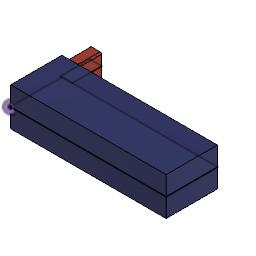
LiPo (Autodesk Fusion 360 design; units mm, degrees)
part number: 2026-02-11-13-17-56-255
Autodesk Fusion 360 part; units mm, degrees
sketch "Sketch1" plane through (0, 0, 0) normal (0, 0, 1) x (1, 0, 0)
  line L0 (0, 0) -> (106, 0)
  line L1 (106, 0) -> (106, 35)
  line L2 (106, 35) -> (0, 35)
  line L3 (0, 35) -> (0, 0)
  line L4 (-1, 35) -> (7, 35)
  line L5 (7, 35) -> (7, 55)
  line L6 (7, 55) -> (-1, 55)
  line L7 (-1, 55) -> (-1, 35)
  dimension "d1" = 106
  dimension "d2" = 35
  dimension "d3" = 8
  dimension "d4" = 20
  dimension "d5" = 1
  constraint horizontal L0
  constraint vertical L1
  constraint horizontal L2
  constraint vertical L3
  constraint coincident L0.start L3.end
  constraint horizontal L4
  constraint vertical L5
  constraint horizontal L6
  constraint vertical L7
  constraint collinear L2 L4
  measures "d1" distance of L0.start L0.end
  measures "d2" distance of L0.start L2.end
  measures "d3" distance of L4.start L4.end
  measures "d4" distance of L4.start L6.end
  measures "d5" distance of L3 L4.start
extrude "Extrude1" add sketch "Sketch1" along normal mid plane 26 contours L0 L1 L2 L3 L4
extrude "Extrude2" add sketch "Sketch1" along normal mid plane 16 contours L2 L4 L5 L6 L7
fillet "Fillet1" radius 1 4 edges at (7, 45, 8) (-1, 45, 8) (-1, 45, -8) (7, 45, -8)
